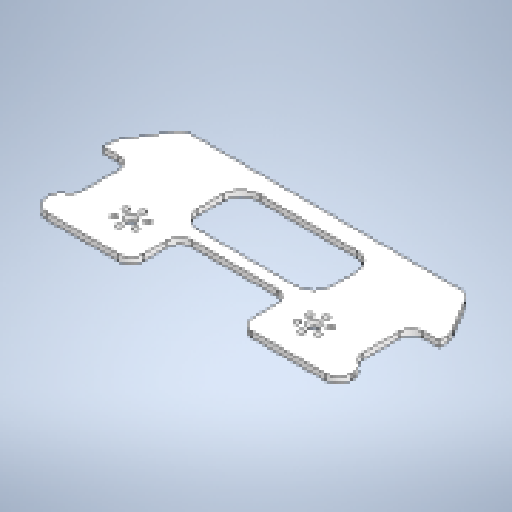
# Autodesk Inventor part: Top Plate
Saved by Autodesk Inventor 2023.2 (Build 272271000, 271)
## iProperties
Created: 2023-06-29
Part Number: Top Plate
Material: UHMW, White
Document SubType Name: Modeling
Designer: Nathan Cai
Mass: 25.5209 g
Surface Area: 194.944 cm^2
Volume: 27.1499 cm^3
Density: 0.94 g/cm^3
Appearance: Smooth - White
Author: Nathan Cai
Autodesk Inventor part; units mm, degrees
ref_plane "YZ Plane" through (0, 0, 0) normal (1, 0, 0) x (0, 1, 0)
ref_plane "XZ Plane" through (0, 0, 0) normal (0, 1, 0) x (-1, 0, 0)
ref_plane "XY Plane" through (0, 0, 0) normal (0, 0, 1) x (1, 0, 0)
sketch "Sketch1" plane through (0, 0, 0) normal (0, 1, 0) x (-1, 0, 0)
  line L0 (-92.075, 39.6875) -> (92.075, 39.6875)
  line L1 (92.075, 39.6875) -> (92.075, -39.6875)
  line L2 (92.075, -39.6875) -> (-92.075, -39.6875)
  line L3 (-92.075, -39.6875) -> (-92.075, 39.6875)
  line L4 (-92.075, 39.6875) -> (92.075, -39.6875) construction
  line L5 (92.075, 39.6875) -> (-92.075, -39.6875) construction
  line L6 (-28.575, 65.0875) -> (28.575, 65.0875)
  line L7 (28.575, 65.0875) -> (28.575, 14.2875)
  line L8 (28.575, 14.2875) -> (-28.575, 14.2875)
  line L9 (-28.575, 14.2875) -> (-28.575, 65.0875)
  line L10 (-28.575, 65.0875) -> (28.575, 14.2875) construction
  line L11 (28.575, 65.0875) -> (-28.575, 14.2875) construction
  line L12 (0, 14.2875) -> (0, -39.6875) construction
  line L13 (-92.075, 26.9875) -> (-73.025, 26.9875)
  line L14 (-73.025, 26.9875) -> (-73.025, -4.7625)
  line L15 (-73.025, -4.7625) -> (-92.075, -4.7625)
  line L16 (-92.075, -4.7625) -> (-92.075, 26.9875)
  line L17 (-92.075, 26.9875) -> (-79.375, 26.9875)
  line L18 (-79.375, 26.9875) -> (-79.375, 39.6875)
  line L19 (-79.375, 39.6875) -> (-92.075, 39.6875)
  line L20 (-92.075, 39.6875) -> (-92.075, 26.9875)
  line L21 (92.075, 26.9875) -> (73.025, 26.9875)
  line L22 (73.025, 26.9875) -> (73.025, -4.7625)
  line L23 (73.025, -4.7625) -> (92.075, -4.7625)
  line L24 (92.075, -4.7625) -> (92.075, 26.9875)
  line L25 (92.075, 26.9875) -> (79.375, 26.9875)
  line L26 (79.375, 26.9875) -> (79.375, 39.6875)
  line L27 (79.375, 39.6875) -> (92.075, 39.6875)
  line L28 (92.075, 39.6875) -> (92.075, 26.9875)
  line L29 (-92.075, -39.6875) -> (-76.2, -39.6875)
  line L30 (-76.2, -39.6875) -> (-76.2, -26.9875)
  line L31 (-76.2, -26.9875) -> (-92.075, -26.9875) construction
  line L32 (-92.075, -26.9875) -> (-92.075, -39.6875)
  line L33 (-76.2, -39.6875) -> (-69.85, -39.6875)
  line L34 (-69.85, -39.6875) -> (-69.85, -33.3375)
  line L35 (-69.85, -33.3375) -> (-76.2, -33.3375) construction
  line L36 (-76.2, -33.3375) -> (-76.2, -39.6875)
  line L37 (-76.2, -33.3375) -> (-92.075, -26.9875)
  line L38 (-76.2, -33.3375) -> (-69.85, -39.6875)
  line L39 (92.075, -39.6875) -> (76.2, -39.6875)
  line L40 (76.2, -39.6875) -> (76.2, -26.9875)
  line L41 (76.2, -26.9875) -> (92.075, -26.9875) construction
  line L42 (92.075, -26.9875) -> (92.075, -39.6875)
  line L43 (76.2, -39.6875) -> (69.85, -39.6875)
  line L44 (69.85, -39.6875) -> (69.85, -33.3375)
  line L45 (69.85, -33.3375) -> (76.2, -33.3375) construction
  line L46 (76.2, -33.3375) -> (76.2, -39.6875)
  line L47 (76.2, -33.3375) -> (92.075, -26.9875)
  line L48 (76.2, -33.3375) -> (69.85, -39.6875)
  line L49 (-34.925, 7.9375) -> (34.925, 7.9375)
  line L50 (34.925, 7.9375) -> (34.925, -23.8125)
  line L51 (34.925, -23.8125) -> (-34.925, -23.8125)
  line L52 (-34.925, -23.8125) -> (-34.925, 7.9375)
  line L53 (-34.925, 7.9375) -> (34.925, -23.8125) construction
  line L54 (34.925, 7.9375) -> (-34.925, -23.8125) construction
  line L55 (-87.3125, -4.7625) -> (-87.3125, -39.6875)
  line L56 (-69.85, -39.6875) -> (-87.3125, -11.1125)
  line L57 (87.3125, -4.7625) -> (87.3125, -39.6875)
  line L58 (69.85, -39.6875) -> (87.3125, -11.1125)
  line L59 (92.075, -33.3375) -> (-92.075, -33.3375)
  point P0 (0, 0)
  point P1 (0, 39.6875)
  point P2 (28.575, 39.6875)
  point P3 (-28.575, 39.6875)
  point P4 (0, -7.9375)
  point P5 (-73.7306, -33.3375)
  point P6 (73.7306, -33.3375)
  dimension "d0" = 184.15
  dimension "d1" = 79.375
  dimension "d4" = 57.15
  dimension "d6" = 25.4
  dimension "d7" = 31.75
  dimension "d8" = 19.05
  dimension "d9" = 12.7
  dimension "d10" = 12.7
  dimension "d11" = 15.875
  dimension "d12" = 12.7
  dimension "d13" = 6.35
  dimension "d14" = 6.35
  dimension "d16" = 69.85
  dimension "d17" = 31.75
  dimension "d18" = 15.875
  dimension "d20" = 4.7625
  dimension "d21" = 6.35
  constraints: 120 end point, 17 symmetric about line, 14 parallel, 11 midpoint, 8 perpendicular, 7 horizontal, 7 point on line
  measures "d0" distance of L1.end L2.end
  measures "d1" distance of L0.end L1.end
  measures "d4" distance of L7.end L8.end
  measures "d6" distance between parallel lines of L0 L8
  measures "d7" distance of L13.end L14.end
  measures "d8" distance between parallel lines of L3 L14
  measures "d9" distance between parallel lines of L0 L13
  measures "d10" distance of L19.end L18.end
  measures "d11" distance of L31.end L30.end
  measures "d12" distance of L30.end L29.end
  measures "d13" distance of L35.end L34.end
  measures "d14" distance of L34.end L33.end
  measures "d16" distance of L50.end L51.end
  measures "d17" distance of L49.end L50.end
  measures "d18" distance between parallel lines of L2 L51
  measures "d20" distance between parallel lines of L3 L55
  measures "d21" distance from line of L15 L56.end
extrude "Extrusion1" add sketch "Sketch1" along normal blind 3.175 contours L0 L9 L8 L7 L26 L21 L22 L23 L57 L58 L59 L56 L55 L15 L14 L13 L18
fillet "Fillet1" radius 6.35 16 edges at (79.375, 1.5875, 39.6875) (79.375, 1.5875, 26.9875) (-79.375, 1.5875, 39.6875) (-79.375, 1.5875, 26.9875) (-73.025, 1.5875, 26.9875) (-73.025, 1.5875, -4.7625) (73.025, 1.5875, 26.9875) (73.025, 1.5875, -4.7625) (28.575, 1.5875, 39.6875) (-28.575, 1.5875, 39.6875) (28.575, 1.5875, 14.2875) (-28.575, 1.5875, 14.2875) (87.3125, 1.5875, -11.1125) (-87.3125, 1.5875, -11.1125) (73.7306, 1.5875, -33.3375) (-73.7306, 1.5875, -33.3375)
fillet "Fillet2" radius 3.175 4 edges at (34.925, 1.5875, 7.9375) (-34.925, 1.5875, 7.9375) (-34.925, 1.5875, -23.8125) (34.925, 1.5875, -23.8125)
sketch "Sketch2" plane through (0, 3.175, 0) normal (0, 1, 0) x (1, 0, 0)
  line L0 (0, 0) -> (0, 39.6875) construction
  line L1 (66.2887, 39.6875) -> (-66.2887, 39.6875) projected
  circle A0 centre (-44.45, -20.6375) radius 3.175
  circle A1 centre (-44.45, -20.6375) radius 6.35 construction
  line L2 (-44.45, -20.6375) -> (-44.45, -26.9875) construction
  circle A2 centre (-44.45, -26.9875) radius 1.5875
  circle A3 centre (-38.9507, -23.8125) radius 1.5875
  circle A4 centre (-38.9507, -17.4625) radius 1.5875
  circle A5 centre (-44.45, -14.2875) radius 1.5875
  circle A6 centre (-49.9493, -17.4625) radius 1.5875
  circle A7 centre (-49.9493, -23.8125) radius 1.5875
  circle A8 centre (-44.45, -20.6375) radius 9.525 construction
  line L3 (-28.575, -33.3375) -> (-28.575, -20.6375) projected
  line L4 (-73.025, -39.6875) -> (-34.925, -39.6875) projected
  circle A9 centre (44.45, -20.6375) radius 3.175
  circle A10 centre (44.45, -20.6375) radius 6.35 construction
  line L5 (44.45, -20.6375) -> (44.45, -26.9875) construction
  circle A11 centre (44.45, -26.9875) radius 1.5875
  circle A12 centre (38.9507, -23.8125) radius 1.5875
  circle A13 centre (38.9507, -17.4625) radius 1.5875
  circle A14 centre (44.45, -14.2875) radius 1.5875
  circle A15 centre (49.9493, -17.4625) radius 1.5875
  circle A16 centre (49.9493, -23.8125) radius 1.5875
  circle A17 centre (44.45, -20.6375) radius 9.525 construction
  dimension "d23" = 12.7
  dimension "d22" = 6.35
  dimension "d24" = 3.175
  dimension "d27" = 360
  dimension "d29" = 19.05
  dimension "d30" = 15.875
  dimension "d31" = 19.05
  constraints: 16 centre point, 10 symmetric about line, 6 coincident, 6 end point, 2 vertical, 2 vertical alignment, 1 midpoint, 25 other
  measures "d22" diameter of A0
  measures "d24" diameter of A2
  measures "d29" diameter of A8
  measures "d30" distance from line of L3 A8.centre
  measures "d31" distance from line of L4 A8.centre
extrude "Extrusion2" cut sketch "Sketch2" against normal blind 3.175
body "Solid1"
